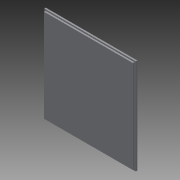
# Autodesk Inventor part: Lid
Saved by Autodesk Inventor 2014 SP1 (Build 180222100, 222)
## iProperties
Created: 2014-11-16
Part Number: Lid
Material: Generic
Document SubType Name: Modeling
Designer: Alex
Density: 1 g/cm^3
Appearance: Default
Author: Alex
Autodesk Inventor part; units mm, degrees
ref_plane "YZ Plane" through (0, 0, 0) normal (1, 0, 0) x (0, 1, 0)
ref_plane "XZ Plane" through (0, 0, 0) normal (0, 1, 0) x (-1, 0, 0)
ref_plane "XY Plane" through (0, 0, 0) normal (0, 0, 1) x (1, 0, 0)
sketch "Sketch1" plane through (0, 0, 0) normal (0, 1, 0) x (-1, 0, 0)
  line L0 (0, 0) -> (116, 0)
  line L1 (116, 0) -> (116, 121)
  line L2 (116, 121) -> (0, 121)
  line L3 (0, 121) -> (0, 0)
  dimension "d0" = 116
  dimension "d1" = 121
  constraints: 8 end point, 2 parallel, 1 horizontal, 1 perpendicular
  measures "d0" distance of L2.end L1.end
  measures "d1" distance of L1.end L0.end
extrude "Extrusion1" add sketch "Sketch1" along normal blind 2
sketch "Sketch2" plane through (0, 2, 0) normal (0, 1, 0) x (1, 0, 0)
  line L0 (1.75, 0) -> (1.75, 1.75)
  line L1 (1.75, 1.75) -> (0, 1.75)
  line L2 (-117.75, -121) -> (-117.75, -122.75)
  line L3 (-117.75, -122.75) -> (-116, -122.75)
  line L4 (-117.75, -122.75) -> (1.75, -122.75)
  line L5 (1.75, -122.75) -> (1.75, 1.75)
  line L6 (1.75, 1.75) -> (-117.75, 1.75)
  line L7 (-117.75, 1.75) -> (-117.75, -122.75)
  dimension "d4" = 1.75
  dimension "d5" = 1.75
  dimension "d6" = 1.75
  dimension "d7" = 1.75
  constraints: 16 end point, 2 parallel, 1 horizontal, 1 perpendicular
  measures "d4" distance of L1.end L0.end
  measures "d5" distance of L0.end L0.start
  measures "d6" distance of L3.end L2.end
  measures "d7" distance of L2.end L2.start
extrude "Extrusion2" add sketch "Sketch2" along normal blind 2
body "Solid1"
